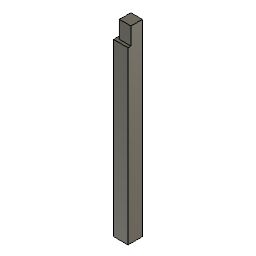
garden-base (Autodesk Fusion 360 archive; units mm, degrees)
design "Leg 50x50"
part number: 2026-07-10-09-27-13-988
Autodesk Fusion 360 part; units mm, degrees
sketch "Sketch1" plane through (0, 0, 0) normal (0, 0, 1) x (1, 0, 0)
  line L0 (0, 0) -> (50, 0)
  line L1 (50, 0) -> (50, 50)
  line L2 (50, 50) -> (0, 50)
  line L3 (0, 50) -> (0, 0)
  dimension "d1" = 50
  dimension "d2" = 50
  constraint horizontal L0
  constraint vertical L1
  constraint horizontal L2
  constraint vertical L3
  constraint coincident L0.start L3.end
  measures "d1" distance of L0.start L0.end
  measures "d2" distance of L0.start L2.end
extrude "Extrude1" add sketch "Sketch1" along normal blind 650
sketch "Sketch2" plane through (0, 0, 650) normal (0, 0, 1) x (-1, 0, 0)
  line L0 (0, -50) -> (0, 0)
  line L1 (0, 0) -> (-50, 0)
  line L2 (-50, 0) -> (-50, -50)
  line L3 (-50, -50) -> (0, -50)
  line L4 (0, -50) -> (-10, -50)
  line L5 (-10, -50) -> (-10, 0)
  line L6 (-10, 0) -> (0, 0)
  line L7 (0, 0) -> (0, -50)
  line L8 (-50, 0) -> (0, 0)
  line L9 (0, 0) -> (0, -10)
  line L10 (0, -10) -> (-50, -10)
  line L11 (-50, -10) -> (-50, 0)
  dimension "d5" = 10
  dimension "d6" = 50
  dimension "d7" = 50
  dimension "d8" = 10
  constraint horizontal L4
  constraint vertical L5
  constraint horizontal L6
  constraint vertical L7
  constraint coincident L0.start L3.end
  constraint horizontal L8
  constraint vertical L9
  constraint horizontal L10
  constraint vertical L11
  constraint coincident L1.end L2.start
  measures "d5" distance of L0.start L4.end
  measures "d6" distance of L0.start L0.end
  measures "d7" distance of L1.end L0.end
  measures "d8" distance of L1.end L10.end
extrude "Extrude2" cut sketch "Sketch2" against normal blind 60 contours L0 L3 L4 L5 L7 L10 | L0 L1 L5 L6 L7 L8 L9 L10 | L1 L2 L5 L8 L10 L11

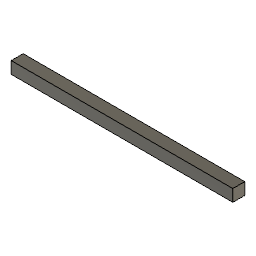
design "Long Rail 50X50"
part number: 2026-07-10-09-30-41-877
Autodesk Fusion 360 part; units mm, degrees
sketch "Sketch1" plane through (0, 0, 0) normal (1, 0, 0) x (0, 1, 0)
  line L0 (0, 0) -> (50, 0)
  line L1 (50, 0) -> (50, 50)
  line L2 (50, 50) -> (0, 50)
  line L3 (0, 50) -> (0, 0)
  dimension "d1" = 50
  dimension "d2" = 50
  constraint horizontal L0
  constraint vertical L1
  constraint horizontal L2
  constraint vertical L3
  constraint coincident L0.start L3.end
  measures "d1" distance of L0.start L0.end
  measures "d2" distance of L0.start L2.end
extrude "Extrude1" add sketch "Sketch1" along normal blind 920

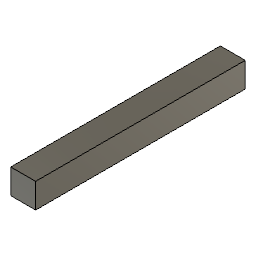
design "Short Rail Bottom 50x50"
part number: 2026-07-10-09-42-50-954
Autodesk Fusion 360 part; units mm, degrees
sketch "Sketch1" plane through (0, 0, 0) normal (0, 1, 0) x (1, 0, 0)
  line L0 (0, 0) -> (50, 0)
  line L1 (50, 0) -> (50, -50)
  line L2 (50, -50) -> (0, -50)
  line L3 (0, -50) -> (0, 0)
  dimension "d1" = 50
  dimension "d2" = 50
  constraint horizontal L0
  constraint vertical L1
  constraint horizontal L2
  constraint vertical L3
  constraint coincident L0.start L3.end
  measures "d1" distance of L0.start L0.end
  measures "d2" distance of L0.start L2.end
extrude "Extrude1" add sketch "Sketch1" along normal blind 420

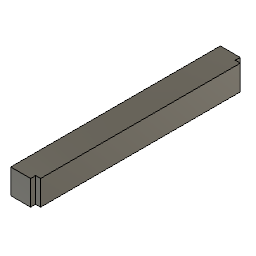
design "Short Rail Top 50x50"
part number: 2026-07-10-09-36-59-418
Autodesk Fusion 360 part; units mm, degrees
sketch "Sketch1" plane through (0, 0, 0) normal (0, 1, 0) x (1, 0, 0)
  line L0 (0, 0) -> (50, 0)
  line L1 (50, 0) -> (50, -50)
  line L2 (50, -50) -> (0, -50)
  line L3 (0, -50) -> (0, 0)
  dimension "d1" = 50
  dimension "d2" = 50
  constraint horizontal L0
  constraint vertical L1
  constraint horizontal L2
  constraint vertical L3
  constraint coincident L0.start L3.end
  measures "d1" distance of L0.start L0.end
  measures "d2" distance of L0.start L2.end
extrude "Extrude1" add sketch "Sketch1" along normal blind 420
sketch "Sketch2" plane through (0, 0, 50) normal (0, 0, 1) x (-1, 0, 0)
  line L0 (0, 0) -> (-50, 0)
  line L1 (-50, 0) -> (-50, -420)
  line L2 (-50, -420) -> (0, -420)
  line L3 (0, -420) -> (0, 0)
  line L4 (-50, 0) -> (-40, 0)
  line L5 (-40, 0) -> (-40, -10)
  line L6 (-40, -10) -> (-50, -10)
  line L7 (-50, -10) -> (-50, 0)
  dimension "d5" = 10
  dimension "d6" = 10
  constraint horizontal L4
  constraint vertical L5
  constraint horizontal L6
  constraint vertical L7
  constraint coincident L0.end L1.start
  measures "d5" distance of L0.end L4.end
  measures "d6" distance of L0.end L6.end
extrude "Extrude2" cut sketch "Sketch2" against normal blind 50 contours L0 L1 L4 L5 L6 L7
sketch "Sketch3" plane through (0, 0, 50) normal (0, 0, 1) x (-1, 0, 0)
  line L0 (-40, -10) -> (-50, -10)
  line L1 (-50, -10) -> (-50, -420)
  line L2 (-50, -420) -> (0, -420)
  line L3 (0, -420) -> (0, 0)
  line L4 (0, 0) -> (-40, 0)
  line L5 (-40, 0) -> (-40, -10)
  line L6 (-50, -420) -> (-40, -420)
  line L7 (-40, -420) -> (-40, -410)
  line L8 (-40, -410) -> (-50, -410)
  line L9 (-50, -410) -> (-50, -420)
  dimension "d9" = 10
  dimension "d10" = 10
  constraint horizontal L6
  constraint vertical L7
  constraint horizontal L8
  constraint vertical L9
  constraint coincident L1.end L2.start
  measures "d9" distance of L1.end L6.end
  measures "d10" distance of L1.end L8.end
extrude "Extrude3" cut sketch "Sketch3" against normal blind 50 contours L1 L2 L6 L7 L8 L9
